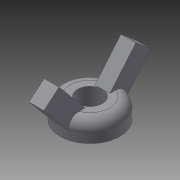
# Autodesk Inventor part: wing_nut
Saved by Autodesk Inventor 2015 (Build 190159000, 159)
## iProperties
Created: 2017-03-25
Part Number: wing_nut
Material: Generic
Document SubType Name: Modeling
Designer: Guy
Density: 1 g/cm^3
Appearance: Default
Author: Guy
Autodesk Inventor part; units mm, degrees
ref_plane "YZ Plane" through (0, 0, 0) normal (1, 0, 0) x (0, 1, 0)
ref_plane "XZ Plane" through (0, 0, 0) normal (0, 1, 0) x (-1, 0, 0)
ref_plane "XY Plane" through (0, 0, 0) normal (0, 0, 1) x (1, 0, 0)
sketch "Sketch1" plane through (0, 0, 0) normal (0, 0, 1) x (1, 0, 0)
  circle A0 centre (0, 0) radius 2.5
  circle A1 centre (0, 0) radius 6
  dimension "d0" = 5
  dimension "d1" = 12
  constraints: 2 centre point, 2 coincident
  measures "d0" diameter of A0
  measures "d1" diameter of A1
extrude "Extrusion1" add sketch "Sketch1" along normal blind 4
fillet "Fillet1" radius 2 1 edges at (-6, 0, 4)
sketch "Sketch2" plane through (0, 0, 0) normal (1, 0, 0) x (0, 1, 0)
  line L0 (1.3011, 2.5712) -> (4.3652, 0)
  line L1 (4.3652, 0) -> (10.7931, 7.6604)
  line L2 (10.7931, 7.6604) -> (7.7289, 10.2316)
  line L3 (7.7289, 10.2316) -> (1.3011, 2.5712)
  line L4 (-1.3011, 2.5712) -> (-4.3652, 0)
  line L5 (-4.3652, 0) -> (-10.7931, 7.6604)
  line L6 (-10.7931, 7.6604) -> (-7.7289, 10.2316)
  line L7 (-7.7289, 10.2316) -> (-1.3011, 2.5712)
  line L8 (-6, 0) -> (6, 0) projected
  line L9 (-2.5, 4) -> (2.5, 4) projected
  point P0 (0, 0)
  dimension "d5" = 50
  dimension "d6" = 50
  dimension "d7" = 4
  dimension "d8" = 4
  dimension "d9" = 10
  dimension "d10" = 10
  constraints: 17 end point, 5 perpendicular, 4 point on line, 1 parallel
  measures "d5" angle of L8 L5
  measures "d6" angle of L8 L1
  measures "d7" distance between parallel lines of L5 L7
  measures "d8" distance between parallel lines of L1 L3
  measures "d9" distance of L6.end L4.start
  measures "d10" distance of L2.end L0.start
extrude "Extrusion2" add sketch "Sketch2" along normal mid plane 3 contours L3 L2 L1 L0 | L5 L6 L7 L4
sketch "Sketch3" plane through (0, 0, 4) normal (0, 0, 1) x (1, 0, 0)
  circle A0 centre (0, 0) radius 2.5
  dimension "d13" = 5
  constraints: 1 centre point, 1 coincident
  measures "d13" diameter of A0
extrude "Extrusion3" cut sketch "Sketch3" against normal through all
body "Solid1"
